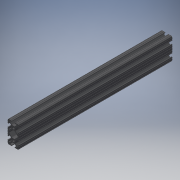
# Autodesk Inventor part: 1020-1-CL
Saved by Autodesk Inventor 2017 (Build 210142000, 142)
## iProperties
Category: PARTsolutions
Company: 8020
Created: 2017-08-20
Part Number: 1020-1-CL
Catalog Web Link: www.cadenas.de
Description: 1020-T-Slotted Profile - 10 Series
Vendor: 8020
Document SubType Name: Modeling
Designer: psAdmin
Manufacturer: 8020
Mass: 12.8943 g
Surface Area: 112.124 cm^2
Volume: 12.8943 cm^3
Density: 1 g/cm^3
Material: Generic
Appearance: PSOLRGB-175-175-175
PSOL_IDENT_0: {$CADENAS_DATA\23d-libs\8020\inch\profiles\10_series\1020.prj},159 {VTYP=3D},{NB=1020-1-CL},{LINA=10
PSOL_IDENT_1: 20-1},{NN=1020},{DATE=03.04.2014 08:24:36},{GEOMDATE=03.04.2014 08:23:00},{VERSION=},{LINEID=10},{LI
PSOL_IDENT_2: NESUBID=-1},{WBVAR=LS,L}  {NB=1020-1-CL},{LINA=1020-1},{KT=DUMMY},{PN=1020-1},{SERIES=1020},{MAT=610
PSOL_IDENT_3: 5-T5 Aluminum},{FIN=Clear Anodize},{LS=-CL},{L=1.000},{LALG=[1:242/0.005]},{W=.9212},{MIX=.3078},{MI
PSOL_IDENT_4: Y=.0833},{EA=.7914}
NN: 1020
NT: T-Slotted Profile - 10 Series
NB: 1020-1-CL
NBSYN: $PN.$LS.
LINA: 1020-1
PN: 1020-1
SERIES: 1020
MAT: 6105-T5 Aluminum
FIN: Clear Anodize
LS: Custom Length
L: 1.000
W: .9212
MIX: .3078
MIY: .0833
EA: .7914
SUPPLIER: 8020
ARTICLENO: 1020-1-CL
BOMINFO: 1020-1
CREATOR: CADENAS GmbH
Title: 1020-1
Author: Cadenas PARTsolutions
Comments: T-Slotted Profile - 10 Series
Autodesk Inventor part; units mm, degrees
ref_plane "YZ Plane" through (0, 0, 0) normal (1, 0, 0) x (0, 1, 0)
ref_plane "XZ Plane" through (0, 0, 0) normal (0, 1, 0) x (-1, 0, 0)
ref_plane "XY Plane" through (0, 0, 0) normal (0, 0, 1) x (1, 0, 0)
sketch "Sketch_1" plane through (0, 0, 0) normal (0, 0, 1) x (1, 0, 0)
  line L0 (-12.7, 34.9504) -> (-12.7, 31.7246)
  arc A0 (-12.7, 30.7086) -> (-12.7, 31.7246) centre (-12.7, 31.2166) ccw
  line L1 (-12.7, 30.7086) -> (-12.7, 29.7023)
  arc A1 (-12.7, 29.7023) -> (-10.4902, 29.7023) centre (-11.5951, 29.7023) ccw
  line L2 (-10.4902, 29.7023) -> (-10.4902, 31.8748)
  arc A2 (-8.7558, 32.5932) -> (-10.4902, 31.8748) centre (-9.4742, 31.8748) ccw
  line L3 (-8.7558, 32.5932) -> (-5.4384, 29.2759)
  arc A3 (-4.5085, 27.0308) -> (-5.4384, 29.2759) centre (-7.6835, 27.0308) ccw
  line L4 (-4.5085, 27.0308) -> (-4.5085, 23.7692)
  arc A4 (-5.4384, 21.5241) -> (-4.5085, 23.7692) centre (-7.6835, 23.7692) ccw
  line L5 (-5.4384, 21.5241) -> (-8.7558, 18.2068)
  arc A5 (-10.4902, 18.9252) -> (-8.7558, 18.2068) centre (-9.4742, 18.9252) ccw
  line L6 (-10.4902, 18.9252) -> (-10.4902, 21.0977)
  arc A6 (-10.4902, 21.0977) -> (-12.7, 21.0977) centre (-11.5951, 21.0977) ccw
  line L7 (-12.7, 21.0977) -> (-12.7, 20.0914)
  arc A7 (-12.7, 19.0754) -> (-12.7, 20.0914) centre (-12.7, 19.5834) ccw
  line L8 (-12.7, 19.0754) -> (-12.7, 15.8496)
  arc A8 (-12.7, 14.8336) -> (-12.7, 15.8496) centre (-12.7, 15.3416) ccw
  line L9 (-12.7, 14.8336) -> (-12.7, 10.5664)
  arc A9 (-12.7, 9.5504) -> (-12.7, 10.5664) centre (-12.7, 10.0584) ccw
  line L10 (-12.7, 9.5504) -> (-12.7, 6.3246)
  arc A10 (-12.7, 5.3086) -> (-12.7, 6.3246) centre (-12.7, 5.8166) ccw
  line L11 (-12.7, 5.3086) -> (-12.7, 4.3023)
  arc A11 (-12.7, 4.3023) -> (-10.4902, 4.3023) centre (-11.5951, 4.3023) ccw
  line L12 (-10.4902, 4.3023) -> (-10.4902, 6.4748)
  arc A12 (-8.7558, 7.1932) -> (-10.4902, 6.4748) centre (-9.4742, 6.4748) ccw
  line L13 (-8.7558, 7.1932) -> (-5.4384, 3.8759)
  arc A13 (-4.5085, 1.6308) -> (-5.4384, 3.8759) centre (-7.6835, 1.6308) ccw
  line L14 (-4.5085, 1.6308) -> (-4.5085, -1.6308)
  arc A14 (-5.4384, -3.8759) -> (-4.5085, -1.6308) centre (-7.6835, -1.6308) ccw
  line L15 (-5.4384, -3.8759) -> (-8.7558, -7.1932)
  arc A15 (-10.4902, -6.4748) -> (-8.7558, -7.1932) centre (-9.4742, -6.4748) ccw
  line L16 (-10.4902, -6.4748) -> (-10.4902, -4.3023)
  arc A16 (-10.4902, -4.3023) -> (-12.7, -4.3023) centre (-11.5951, -4.3023) ccw
  line L17 (-12.7, -4.3023) -> (-12.7, -5.3086)
  arc A17 (-12.7, -6.3246) -> (-12.7, -5.3086) centre (-12.7, -5.8166) ccw
  line L18 (-12.7, -6.3246) -> (-12.7, -9.5504)
  arc A18 (-12.7, -10.5791) -> (-12.7, -9.5504) centre (-12.7064, -10.0648) ccw
  arc A19 (-12.7, -10.5791) -> (-10.5791, -12.7) centre (-10.5918, -10.5918) ccw
  arc A20 (-9.5504, -12.7) -> (-10.5791, -12.7) centre (-10.0648, -12.7064) ccw
  line L19 (-9.5504, -12.7) -> (-6.3246, -12.7)
  arc A21 (-5.3086, -12.7) -> (-6.3246, -12.7) centre (-5.8166, -12.7) ccw
  line L20 (-5.3086, -12.7) -> (-4.3023, -12.7)
  arc A22 (-4.3023, -12.7) -> (-4.3023, -10.4902) centre (-4.3023, -11.5951) ccw
  line L21 (-4.3023, -10.4902) -> (-6.4748, -10.4902)
  arc A23 (-7.1932, -8.7558) -> (-6.4748, -10.4902) centre (-6.4748, -9.4742) ccw
  line L22 (-7.1932, -8.7558) -> (-3.8759, -5.4384)
  arc A24 (-1.6308, -4.5085) -> (-3.8759, -5.4384) centre (-1.6308, -7.6835) ccw
  line L23 (-1.6308, -4.5085) -> (1.6308, -4.5085)
  arc A25 (3.8759, -5.4384) -> (1.6308, -4.5085) centre (1.6308, -7.6835) ccw
  line L24 (3.8759, -5.4384) -> (7.1932, -8.7558)
  arc A26 (6.4748, -10.4902) -> (7.1932, -8.7558) centre (6.4748, -9.4742) ccw
  line L25 (6.4748, -10.4902) -> (4.3023, -10.4902)
  arc A27 (4.3023, -10.4902) -> (4.3023, -12.7) centre (4.3023, -11.5951) ccw
  line L26 (4.3023, -12.7) -> (5.3086, -12.7)
  arc A28 (6.3246, -12.7) -> (5.3086, -12.7) centre (5.8166, -12.7) ccw
  line L27 (6.3246, -12.7) -> (9.5504, -12.7)
  arc A29 (10.5791, -12.7) -> (9.5504, -12.7) centre (10.0648, -12.7064) ccw
  arc A30 (10.5791, -12.7) -> (12.7, -10.5791) centre (10.5918, -10.5918) ccw
  arc A31 (12.7, -9.5504) -> (12.7, -10.5791) centre (12.7064, -10.0648) ccw
  line L28 (12.7, -9.5504) -> (12.7, -6.3246)
  arc A32 (12.7, -5.3086) -> (12.7, -6.3246) centre (12.7, -5.8166) ccw
  line L29 (12.7, -5.3086) -> (12.7, -4.3023)
  arc A33 (12.7, -4.3023) -> (10.4902, -4.3023) centre (11.5951, -4.3023) ccw
  line L30 (10.4902, -4.3023) -> (10.4902, -6.4748)
  arc A34 (8.7558, -7.1932) -> (10.4902, -6.4748) centre (9.4742, -6.4748) ccw
  line L31 (8.7558, -7.1932) -> (5.4384, -3.8759)
  arc A35 (4.5085, -1.6308) -> (5.4384, -3.8759) centre (7.6835, -1.6308) ccw
  line L32 (4.5085, -1.6308) -> (4.5085, 1.6308)
  arc A36 (5.4384, 3.8759) -> (4.5085, 1.6308) centre (7.6835, 1.6308) ccw
  line L33 (5.4384, 3.8759) -> (8.7558, 7.1932)
  arc A37 (10.4902, 6.4748) -> (8.7558, 7.1932) centre (9.4742, 6.4748) ccw
  line L34 (10.4902, 6.4748) -> (10.4902, 4.3023)
  arc A38 (10.4902, 4.3023) -> (12.7, 4.3023) centre (11.5951, 4.3023) ccw
  line L35 (12.7, 4.3023) -> (12.7, 5.3086)
  arc A39 (12.7, 6.3246) -> (12.7, 5.3086) centre (12.7, 5.8166) ccw
  line L36 (12.7, 6.3246) -> (12.7, 9.5504)
  arc A40 (12.7, 10.5664) -> (12.7, 9.5504) centre (12.7, 10.0584) ccw
  line L37 (12.7, 10.5664) -> (12.7, 14.8336)
  arc A41 (12.7, 15.8496) -> (12.7, 14.8336) centre (12.7, 15.3416) ccw
  line L38 (12.7, 15.8496) -> (12.7, 19.0754)
  arc A42 (12.7, 20.0914) -> (12.7, 19.0754) centre (12.7, 19.5834) ccw
  line L39 (12.7, 20.0914) -> (12.7, 21.0977)
  arc A43 (12.7, 21.0977) -> (10.4902, 21.0977) centre (11.5951, 21.0977) ccw
  line L40 (10.4902, 21.0977) -> (10.4902, 18.9252)
  arc A44 (8.7558, 18.2068) -> (10.4902, 18.9252) centre (9.4742, 18.9252) ccw
  line L41 (8.7558, 18.2068) -> (5.4384, 21.5241)
  arc A45 (4.5085, 23.7692) -> (5.4384, 21.5241) centre (7.6835, 23.7692) ccw
  line L42 (4.5085, 23.7692) -> (4.5085, 27.0308)
  arc A46 (5.4384, 29.2759) -> (4.5085, 27.0308) centre (7.6835, 27.0308) ccw
  line L43 (5.4384, 29.2759) -> (8.7558, 32.5932)
  arc A47 (10.4902, 31.8748) -> (8.7558, 32.5932) centre (9.4742, 31.8748) ccw
  line L44 (10.4902, 31.8748) -> (10.4902, 29.7023)
  arc A48 (10.4902, 29.7023) -> (12.7, 29.7023) centre (11.5951, 29.7023) ccw
  line L45 (12.7, 29.7023) -> (12.7, 30.7086)
  arc A49 (12.7, 31.7246) -> (12.7, 30.7086) centre (12.7, 31.2166) ccw
  line L46 (12.7, 31.7246) -> (12.7, 34.9504)
  arc A50 (12.7, 35.9791) -> (12.7, 34.9504) centre (12.7064, 35.4648) ccw
  arc A51 (12.7, 35.9791) -> (10.5791, 38.1) centre (10.5918, 35.9918) ccw
  arc A52 (9.5504, 38.1) -> (10.5791, 38.1) centre (10.0648, 38.1063) ccw
  line L47 (9.5504, 38.1) -> (6.3246, 38.1)
  arc A53 (5.3086, 38.1) -> (6.3246, 38.1) centre (5.8166, 38.1) ccw
  line L48 (5.3086, 38.1) -> (4.3023, 38.1)
  arc A54 (4.3023, 38.1) -> (4.3023, 35.8902) centre (4.3023, 36.9951) ccw
  line L49 (4.3023, 35.8902) -> (6.4748, 35.8902)
  arc A55 (7.1932, 34.1558) -> (6.4748, 35.8902) centre (6.4748, 34.8742) ccw
  line L50 (7.1932, 34.1558) -> (3.8759, 30.8384)
  arc A56 (1.6308, 29.9085) -> (3.8759, 30.8384) centre (1.6308, 33.0835) ccw
  line L51 (1.6308, 29.9085) -> (-1.6308, 29.9085)
  arc A57 (-3.8759, 30.8384) -> (-1.6308, 29.9085) centre (-1.6308, 33.0835) ccw
  line L52 (-3.8759, 30.8384) -> (-7.1932, 34.1558)
  arc A58 (-6.4748, 35.8902) -> (-7.1932, 34.1558) centre (-6.4748, 34.8742) ccw
  line L53 (-6.4748, 35.8902) -> (-4.3023, 35.8902)
  arc A59 (-4.3023, 35.8902) -> (-4.3023, 38.1) centre (-4.3023, 36.9951) ccw
  line L54 (-4.3023, 38.1) -> (-5.3086, 38.1)
  arc A60 (-6.3246, 38.1) -> (-5.3086, 38.1) centre (-5.8166, 38.1) ccw
  line L55 (-6.3246, 38.1) -> (-9.5504, 38.1)
  arc A61 (-10.5791, 38.1) -> (-9.5504, 38.1) centre (-10.0648, 38.1063) ccw
  arc A62 (-10.5791, 38.1) -> (-12.7, 35.9791) centre (-10.5918, 35.9918) ccw
  arc A63 (-12.7, 34.9504) -> (-12.7, 35.9791) centre (-12.7064, 35.4648) ccw
  circle A64 centre (0, 0) radius 2.6035
  circle A65 centre (0, 25.4) radius 2.6035
  arc A66 (-10.033, 12.2479) -> (-9.5718, 11.1343) centre (-8.4582, 12.2479) ccw
  line L56 (-9.5718, 11.1343) -> (-3.8759, 5.4384)
  arc A67 (-3.8759, 5.4384) -> (-1.6308, 4.5085) centre (-1.6308, 7.6835) ccw
  line L57 (-1.6308, 4.5085) -> (1.6308, 4.5085)
  arc A68 (1.6308, 4.5085) -> (3.8759, 5.4384) centre (1.6308, 7.6835) ccw
  line L58 (3.8759, 5.4384) -> (9.5718, 11.1343)
  arc A69 (9.5718, 11.1343) -> (10.033, 12.2479) centre (8.4582, 12.2479) ccw
  line L59 (10.033, 12.2479) -> (10.033, 13.1521)
  arc A70 (10.033, 13.1521) -> (9.5718, 14.2657) centre (8.4582, 13.1521) ccw
  line L60 (9.5718, 14.2657) -> (3.8759, 19.9616)
  arc A71 (3.8759, 19.9616) -> (1.6308, 20.8915) centre (1.6308, 17.7165) ccw
  line L61 (1.6308, 20.8915) -> (-1.6308, 20.8915)
  arc A72 (-1.6308, 20.8915) -> (-3.8759, 19.9616) centre (-1.6308, 17.7165) ccw
  line L62 (-3.8759, 19.9616) -> (-9.5718, 14.2657)
  arc A73 (-9.5718, 14.2657) -> (-10.033, 13.1521) centre (-8.4582, 13.1521) ccw
  line L63 (-10.033, 13.1521) -> (-10.033, 12.2479)
  constraints: 144 point on circle, 128 end point, 74 centre point
extrude "Extrusion1" add sketch "Sketch_1" against normal blind 355.6
ref_plane "b1_XY" through (0, -12.7, -12.7) normal (0, 1, 0) x (1, 0, 0)
ref_plane "b1_YZ" through (0, -12.7, -12.7) normal (1, 0, 0) x (0, 0, -1)
ref_plane "b1_ZX" through (0, -12.7, -12.7) normal (0, 0, -1) x (0, 1, 0)
ref_plane "b2_XY" through (0, 38.1, -12.7) normal (0, 1, 0) x (1, 0, 0)
ref_plane "b2_YZ" through (0, 38.1, -12.7) normal (1, 0, 0) x (0, 0, -1)
ref_plane "b2_ZX" through (0, 38.1, -12.7) normal (0, 0, -1) x (0, 1, 0)
ref_plane "profile1020_XY" through (0, 12.7, -12.7) normal (0, 0, 1) x (1, 0, 0)
ref_plane "profile1020_YZ" through (0, 12.7, -12.7) normal (1, 0, 0) x (0, 1, 0)
ref_plane "profile1020_ZX" through (0, 12.7, -12.7) normal (0, 1, 0) x (0, 0, 1)
body "Solid1"
